Autodesk Inventor part; units mm, degrees
(part 2 of 2)
sketch "スケッチ6" plane through (2.9, 8.6756, -79.5656) normal (1, 0, 0) x (0, 0.1072674, -0.9942302)
  arc A0 (-63.7147, -7.4384) -> (-63.7149, 7.2573) centre (-80.0371, -0.0908) ccw projected
  circle A1 centre (-80.87, 51.0359) radius 3.45
  point P0 (-80.0371, -0.0908)
  point P1 (-80.0371, -0.0908)
  dimension "d31" = 6.9
  constraints: 1 centre point
  measures "d31" diameter of A1
extrude "押し出し5" cut sketch "スケッチ6" against normal blind 10
pattern_circular "円形状パターン3" count 6 over 360 about axis through (35.15, 0, 0) along (1, 0, 0) of "押し出し5"
sketch "スケッチ8" plane through (2.9, 8.6756, -79.5656) normal (1, 0, 0) x (0, 0.1072674, -0.9942302)
  circle A0 centre (-80.0371, -0.0908) radius 22.9
  circle A1 centre (-36.1766, 26.1938) radius 3.45 projected
  circle A2 centre (-35.3437, -24.9328) radius 3.45 projected
  circle A3 centre (-79.2043, -51.2174) radius 3.45 projected
  circle A4 centre (-123.8977, -26.3754) radius 3.45 projected
  circle A5 centre (-124.7305, 24.7513) radius 3.45 projected
  circle A6 centre (-80.87, 51.0359) radius 3.45 projected
  arc A7 (-96.3596, 7.2569) -> (-96.3594, -7.4389) centre (-80.0371, -0.0908) ccw projected
  arc A8 (-96.3596, 7.2569) -> (-94.5619, 10.3707) centre (-95.5391, 8.859) ccw projected
  arc A9 (-81.8351, 17.7187) -> (-94.5619, 10.3707) centre (-80.0371, -0.0908) ccw projected
  arc A10 (-81.8351, 17.7187) -> (-78.2397, 17.7188) centre (-80.0374, 17.8092) ccw projected
  arc A11 (-65.5127, 10.3711) -> (-78.2397, 17.7188) centre (-80.0371, -0.0908) ccw projected
  arc A12 (-65.5127, 10.3711) -> (-63.7149, 7.2573) centre (-64.5354, 8.8595) ccw projected
  arc A13 (-63.7147, -7.4384) -> (-63.7149, 7.2573) centre (-80.0371, -0.0908) ccw projected
  arc A14 (-63.7147, -7.4384) -> (-65.5124, -10.5522) centre (-64.5352, -9.0405) ccw projected
  arc A15 (-78.2392, -17.9002) -> (-65.5124, -10.5522) centre (-80.0371, -0.0908) ccw projected
  arc A16 (-78.2392, -17.9002) -> (-81.8346, -17.9003) centre (-80.0369, -17.9908) ccw projected
  arc A17 (-94.5616, -10.5526) -> (-81.8346, -17.9003) centre (-80.0371, -0.0908) ccw projected
  arc A18 (-94.5616, -10.5526) -> (-96.3594, -7.4389) centre (-95.5389, -9.041) ccw projected
  line L0 (-1.0768, -4.9175) -> (1.1501, -3.6267) projected
  arc A19 (1.1501, -3.6267) -> (1.1812, -2.8194) centre (-80.0371, -0.0908) ccw projected
  line L1 (1.1812, -2.8194) -> (-0.9369, -1.3582) projected
  arc A20 (-0.9369, 1.3582) -> (-0.9369, -1.3582) centre (0, 0) ccw projected
  line L2 (-0.9369, 1.3582) -> (1.1751, 2.8151) projected
  arc A21 (1.1751, 2.8151) -> (1.1417, 3.6315) centre (-80.0371, -0.0908) ccw projected
  line L3 (1.1417, 3.6315) -> (-1.0768, 4.9175) projected
  arc A22 (-1.2899, 7.6255) -> (-1.0768, 4.9175) centre (-0.2493, 6.345) ccw projected
  line L4 (-1.2899, 7.6255) -> (0.6902, 9.2346) projected
  arc A23 (0.6902, 9.2346) -> (0.5904, 10.0614) centre (-80.0371, -0.0908) ccw projected
  line L5 (0.5904, 10.0614) -> (-1.7086, 11.1628) projected
  arc A24 (-2.1335, 13.8457) -> (-1.7086, 11.1628) centre (-0.9956, 12.6509) ccw projected
  line L6 (-2.1335, 13.8457) -> (-0.3005, 15.5913) projected
  arc A25 (-0.3005, 15.5913) -> (-0.4698, 16.4293) centre (-80.0371, -0.0908) ccw projected
  line L7 (-0.4698, 16.4293) -> (-2.8284, 17.3393) projected
  arc A26 (-3.4625, 19.9807) -> (-2.8284, 17.3393) centre (-2.2344, 18.8787) ccw projected
  line L8 (-3.4625, 19.9807) -> (-1.7896, 21.8452) projected
  arc A27 (-1.7896, 21.8452) -> (-2.0327, 22.6945) centre (-80.0371, -0.0908) ccw projected
  line L9 (-2.0327, 22.6945) -> (-4.4294, 23.409) projected
  arc A28 (-5.2688, 25.9924) -> (-4.4294, 23.409) centre (-3.9581, 24.9902) ccw projected
  line L10 (-5.2688, 25.9924) -> (-3.7667, 27.9571) projected
  arc A29 (-3.7667, 27.9571) -> (-4.0884, 28.8169) centre (-80.0371, -0.0908) ccw projected
  line L11 (-4.0884, 28.8169) -> (-6.5017, 29.3343) projected
  arc A30 (-7.5412, 31.8439) -> (-6.5017, 29.3343) centre (-6.1559, 30.9476) ccw projected
  line L12 (-7.5412, 31.8439) -> (-6.2182, 33.889) projected
  arc A31 (-6.2182, 33.889) -> (-6.6241, 34.7574) centre (-80.0371, -0.0908) ccw projected
  line L13 (-6.6241, 34.7574) -> (-9.0325, 35.0787) projected
  arc A32 (-10.2657, 37.499) -> (-9.0325, 35.0787) centre (-8.8143, 36.7142) ccw projected
  line L14 (-10.2657, 37.499) -> (-9.1275, 39.6041) projected
  arc A33 (-9.1275, 39.6041) -> (-9.6237, 40.4779) centre (-80.0371, -0.0908) ccw projected
  line L15 (-9.6237, 40.4779) -> (-12.0062, 40.6069) projected
  arc A34 (-13.4255, 42.923) -> (-12.0062, 40.6069) centre (-11.917, 42.2545) ccw projected
  line L16 (-13.4255, 42.923) -> (-12.4752, 45.0673) projected
  arc A35 (-12.4752, 45.0673) -> (-13.068, 45.9418) centre (-80.0371, -0.0908) ccw projected
  line L17 (-13.068, 45.9418) -> (-15.4045, 45.8847) projected
  arc A36 (-17.0011, 48.0823) -> (-15.4045, 45.8847) centre (-15.4448, 47.5342) ccw projected
  line L18 (-17.0011, 48.0823) -> (-16.2394, 50.2452) projected
  arc A37 (-16.2394, 50.2452) -> (-16.9348, 51.1144) centre (-80.0371, -0.0908) ccw projected
  line L19 (-16.9348, 51.1144) -> (-19.2063, 50.8796) projected
  arc A38 (-20.9705, 52.9451) -> (-19.2063, 50.8796) centre (-19.376, 52.5209) ccw projected
  line L20 (-20.9705, 52.9451) -> (-20.3954, 55.1064) projected
  arc A39 (-20.3954, 55.1064) -> (-21.1994, 55.9626) centre (-80.0371, -0.0908) ccw projected
  line L21 (-21.1994, 55.9626) -> (-23.3884, 55.5608) projected
  arc A40 (-25.3092, 57.4816) -> (-23.3884, 55.5608) centre (-23.6863, 57.1837) ccw projected
  line L22 (-25.3092, 57.4816) -> (-24.9164, 59.6216) projected
  arc A41 (-24.9164, 59.6216) -> (-25.8341, 60.4559) centre (-80.0371, -0.0908) ccw projected
  line L23 (-25.8341, 60.4559) -> (-27.9249, 59.8995) projected
  arc A42 (-29.9904, 61.6637) -> (-27.9249, 59.8995) centre (-28.3491, 61.494) ccw projected
  line L24 (-29.9904, 61.6637) -> (-29.7733, 63.7639) projected
  arc A43 (-29.7733, 63.7639) -> (-30.809, 64.5657) centre (-80.0371, -0.0908) ccw projected
  line L25 (-30.809, 64.5657) -> (-32.7877, 63.8689) projected
  arc A44 (-34.9853, 65.4655) -> (-32.7877, 63.8689) centre (-33.3358, 65.4252) ccw projected
  line L26 (-34.9853, 65.4655) -> (-34.9354, 67.5088) projected
  arc A45 (-34.9354, 67.5088) -> (-36.0922, 68.2665) centre (-80.0371, -0.0908) ccw projected
  line L27 (-36.0922, 68.2665) -> (-37.947, 67.4445) projected
  arc A46 (-40.2631, 68.8638) -> (-37.947, 67.4445) centre (-38.6155, 68.953) ccw projected
  line L28 (-40.2631, 68.8638) -> (-40.3698, 70.8343) projected
  arc A47 (-40.3698, 70.8343) -> (-41.6496, 71.5351) centre (-80.0371, -0.0908) ccw projected
  line L29 (-41.6496, 71.5351) -> (-43.371, 70.6043) projected
  arc A48 (-45.7913, 71.8375) -> (-43.371, 70.6043) centre (-44.1558, 72.0557) ccw projected
  line L30 (-45.7913, 71.8375) -> (-46.0427, 73.7214) projected
  arc A49 (-46.0427, 73.7214) -> (-47.4454, 74.3514) centre (-80.0371, -0.0908) ccw projected
  line L31 (-47.4454, 74.3514) -> (-49.0261, 73.3288) projected
  arc A50 (-51.5357, 74.3683) -> (-49.0261, 73.3288) centre (-49.9224, 74.7141) ccw projected
  line L32 (-51.5357, 74.3683) -> (-51.9185, 76.1536) projected
  arc A51 (-51.9185, 76.1536) -> (-53.4424, 76.6985) centre (-80.0371, -0.0908) ccw projected
  line L33 (-53.4424, 76.6985) -> (-54.8776, 75.6012) projected
  arc A52 (-57.461, 76.4406) -> (-54.8776, 75.6012) centre (-55.8798, 76.9119) ccw projected
  line L34 (-57.461, 76.4406) -> (-57.9609, 78.1173) projected
  arc A53 (-57.9609, 78.1173) -> (-59.6024, 78.5622) centre (-80.0371, -0.0908) ccw projected
  line L35 (-59.6024, 78.5622) -> (-60.8893, 77.4075) projected
  arc A54 (-63.5307, 78.0416) -> (-60.8893, 77.4075) centre (-61.9913, 78.6356) ccw projected
  line L36 (-63.5307, 78.0416) -> (-64.1327, 79.6019) projected
  arc A55 (-64.1327, 79.6019) -> (-65.886, 79.9318) centre (-80.0371, -0.0908) ccw projected
  line L37 (-65.886, 79.9318) -> (-67.0243, 78.7365) projected
  arc A56 (-69.7072, 79.1614) -> (-67.0243, 78.7365) centre (-68.2191, 79.8744) ccw projected
  line L38 (-69.7072, 79.1614) -> (-70.3962, 80.5995) projected
  arc A57 (-70.3962, 80.5995) -> (-72.2514, 80.7996) centre (-80.0371, -0.0908) ccw projected
  line L39 (-72.2514, 80.7996) -> (-73.2346, 79.5639) projected
  arc A58 (-75.9446, 79.749) -> (-73.2346, 79.5639) centre (-74.5257, 80.5912) ccw projected
  line L40 (-75.9446, 79.749) -> (-76.7506, 81.1069) projected
  arc A59 (-76.7506, 81.1069) -> (-78.622, 81.1611) centre (-80.0371, -0.0908) ccw projected
  line L41 (-78.622, 81.1611) -> (-79.5052, 79.8521) projected
  arc A60 (-82.2214, 79.824) -> (-79.5052, 79.8521) centre (-80.873, 80.7749) ccw projected
  line L42 (-82.2214, 79.824) -> (-83.1315, 81.1145) projected
  arc A61 (-83.1315, 81.1145) -> (-85.0013, 81.0217) centre (-80.0371, -0.0908) ccw projected
  line L43 (-85.0013, 81.0217) -> (-85.7791, 79.6474) projected
  arc A62 (-88.4847, 79.4063) -> (-85.7791, 79.6474) centre (-87.215, 80.4601) ccw projected
  line L44 (-88.4847, 79.4063) -> (-89.4932, 80.6214) projected
  arc A63 (-89.4932, 80.6214) -> (-91.35, 80.3821) centre (-80.0371, -0.0908) ccw projected
  line L45 (-91.35, 80.3821) -> (-92.0175, 78.9511) projected
  arc A64 (-94.6959, 78.4984) -> (-92.0175, 78.9511) centre (-93.5129, 79.6486) ccw projected
  line L46 (-94.6959, 78.4984) -> (-95.7967, 79.6307) projected
  arc A65 (-95.7967, 79.6307) -> (-97.629, 79.2465) centre (-80.0371, -0.0908) ccw projected
  line L47 (-97.629, 79.2465) -> (-98.1822, 77.7674) projected
  arc A66 (-100.8168, 77.106) -> (-98.1822, 77.7674) centre (-99.7276, 78.3455) ccw projected
  line L48 (-100.8168, 77.106) -> (-102.0029, 78.1484) projected
  arc A67 (-102.0029, 78.1484) -> (-103.7995, 77.6217) centre (-80.0371, -0.0908) ccw projected
  line L49 (-103.7995, 77.6217) -> (-104.2349, 76.1038) projected
  arc A68 (-106.8095, 75.2377) -> (-104.2349, 76.1038) centre (-105.8209, 76.5588) ccw projected
  line L50 (-106.8095, 75.2377) -> (-108.0738, 76.1838) projected
  arc A69 (-108.0738, 76.1838) -> (-109.8235, 75.5177) centre (-80.0371, -0.0908) ccw projected
  line L51 (-109.8235, 75.5177) -> (-110.1385, 73.9704) projected
  arc A70 (-112.6372, 72.905) -> (-110.1385, 73.9704) centre (-111.7553, 74.2995) ccw projected
  line L52 (-112.6372, 72.905) -> (-113.9718, 73.749) projected
  arc A71 (-113.9718, 73.749) -> (-115.6638, 72.9476) centre (-80.0371, -0.0908) ccw projected
  line L53 (-115.6638, 72.9476) -> (-115.8564, 71.3803) projected
  arc A72 (-118.2639, 70.1222) -> (-115.8564, 71.3803) centre (-117.4941, 71.5816) ccw projected
  line L54 (-118.2639, 70.1222) -> (-119.6606, 70.8589) projected
  arc A73 (-119.6606, 70.8589) -> (-121.2845, 69.9273) centre (-80.0371, -0.0908) ccw projected
  line L55 (-121.2845, 69.9273) -> (-121.3536, 68.3497) projected
  arc A74 (-123.6549, 66.9065) -> (-121.3536, 68.3497) centre (-123.002, 68.4219) ccw projected
  line L56 (-123.6549, 66.9065) -> (-125.1051, 67.5313) projected
  arc A75 (-125.1051, 67.5313) -> (-126.6509, 66.4752) centre (-80.0371, -0.0908) ccw projected
  line L57 (-126.6509, 66.4752) -> (-126.596, 64.897) projected
  arc A76 (-128.777, 63.2778) -> (-126.596, 64.897) centre (-128.245, 64.8397) ccw projected
  line L58 (-128.777, 63.2778) -> (-130.2717, 63.7869) projected
  arc A77 (-130.2717, 63.7869) -> (-131.7299, 62.6127) centre (-80.0371, -0.0908) ccw projected
  line L59 (-131.7299, 62.6127) -> (-131.5514, 61.0437) projected
  arc A78 (-133.5986, 59.2583) -> (-131.5514, 61.0437) centre (-133.1908, 60.8572) ccw projected
  line L60 (-133.5986, 59.2583) -> (-135.1287, 59.6486) projected
  arc A79 (-135.1287, 59.6486) -> (-136.4902, 58.3636) centre (-80.0371, -0.0908) ccw projected
  line L61 (-136.4902, 58.3636) -> (-136.1891, 56.8135) projected
  arc A80 (-138.0899, 54.873) -> (-136.1891, 56.8135) centre (-137.8088, 56.4989) ccw projected
  line L62 (-138.0899, 54.873) -> (-139.6459, 55.142) projected
  arc A81 (-139.6459, 55.142) -> (-140.9025, 53.7542) centre (-80.0371, -0.0908) ccw projected
  line L63 (-140.9025, 53.7542) -> (-140.4807, 52.2325) projected
  arc A82 (-142.2234, 50.1488) -> (-140.4807, 52.2325) centre (-142.0707, 51.7917) ccw projected
  line L64 (-142.2234, 50.1488) -> (-143.7957, 50.2949) projected
  arc A83 (-143.7957, 50.2949) -> (-144.9395, 48.8128) centre (-80.0371, -0.0908) ccw projected
  line L65 (-144.9395, 48.8128) -> (-144.3996, 47.3288) projected
  arc A84 (-145.9734, 45.1149) -> (-144.3996, 47.3288) centre (-145.9501, 46.7647) ccw projected
  line L66 (-145.9734, 45.1149) -> (-147.5524, 45.1371) projected
  arc A85 (-147.5524, 45.1371) -> (-148.5763, 43.5698) centre (-80.0371, -0.0908) ccw projected
  line L67 (-148.5763, 43.5698) -> (-147.9217, 42.1328) projected
  arc A86 (-149.317, 39.8022) -> (-147.9217, 42.1328) centre (-149.4232, 41.4488) ccw projected
  line L68 (-149.317, 39.8022) -> (-150.8928, 39.7005) projected
  arc A87 (-150.8928, 39.7005) -> (-151.7906, 38.0577) centre (-80.0371, -0.0908) ccw projected
  line L69 (-151.7906, 38.0577) -> (-151.0252, 36.6765) projected
  arc A88 (-152.2334, 34.2436) -> (-151.0252, 36.6765) centre (-152.4685, 35.8768) ccw projected
  line L70 (-152.2334, 34.2436) -> (-153.7963, 34.0186) projected
  arc A89 (-153.7963, 34.0186) -> (-154.5625, 32.3104) centre (-80.0371, -0.0908) ccw projected
  line L71 (-154.5625, 32.3104) -> (-153.6911, 30.9935) projected
  arc A90 (-154.7046, 28.4733) -> (-153.6911, 30.9935) centre (-155.0672, 30.083) ccw projected
  line L72 (-154.7046, 28.4733) -> (-156.2452, 28.1264) projected
  arc A91 (-156.2452, 28.1264) -> (-156.8749, 26.3633) centre (-80.0371, -0.0908) ccw projected
  line L73 (-156.8749, 26.3633) -> (-155.9029, 25.1189) projected
  arc A92 (-156.7156, 22.5269) -> (-155.9029, 25.1189) centre (-157.2033, 24.1032) ccw projected
  line L74 (-156.7156, 22.5269) -> (-158.2241, 22.0602) projected
  arc A93 (-158.2241, 22.0602) -> (-158.7136, 20.2532) centre (-80.0371, -0.0908) ccw projected
  line L75 (-158.7136, 20.2532) -> (-157.647, 19.0888) projected
  arc A94 (-158.2538, 16.4411) -> (-157.647, 19.0888) centre (-158.8636, 17.9742) ccw projected
  line L76 (-158.2538, 16.4411) -> (-159.721, 15.8574) projected
  arc A95 (-159.721, 15.8574) -> (-160.0673, 14.0176) centre (-80.0371, -0.0908) ccw projected
  line L77 (-160.0673, 14.0176) -> (-158.9125, 12.9405) projected
  arc A96 (-159.3097, 10.2533) -> (-158.9125, 12.9405) centre (-160.038, 11.7339) ccw projected
  line L78 (-159.3097, 10.2533) -> (-160.7267, 9.5563) projected
  arc A97 (-160.7267, 9.5563) -> (-160.9275, 7.695) centre (-80.0371, -0.0908) ccw projected
  line L79 (-160.9275, 7.695) -> (-159.6918, 6.7118) projected
  arc A98 (-159.8769, 4.0018) -> (-159.6918, 6.7118) centre (-160.7191, 5.4206) ccw projected
  line L80 (-159.8769, 4.0018) -> (-161.2348, 3.1958) projected
  arc A99 (-161.2348, 3.1958) -> (-161.289, 1.3244) centre (-80.0371, -0.0908) ccw projected
  line L81 (-161.289, 1.3244) -> (-159.98, 0.4412) projected
  arc A100 (-159.9519, -2.275) -> (-159.98, 0.4412) centre (-160.9028, -0.9266) ccw projected
  line L82 (-159.9519, -2.275) -> (-161.2424, -3.1851) projected
  arc A101 (-161.2424, -3.1851) -> (-161.1496, -5.0549) centre (-80.0371, -0.0908) ccw projected
  line L83 (-161.1496, -5.0549) -> (-159.7753, -5.8327) projected
  arc A102 (-159.5342, -8.5383) -> (-159.7753, -5.8327) centre (-160.588, -7.2687) ccw projected
  line L84 (-159.5342, -8.5383) -> (-160.7493, -9.5468) projected
  arc A103 (-160.7493, -9.5468) -> (-160.51, -11.4036) centre (-80.0371, -0.0908) ccw projected
  line L85 (-160.51, -11.4036) -> (-159.079, -12.0712) projected
  arc A104 (-158.6263, -14.7495) -> (-159.079, -12.0712) centre (-159.7765, -13.5665) ccw projected
  line L86 (-158.6263, -14.7495) -> (-159.7586, -15.8503) projected
  arc A105 (-159.7586, -15.8503) -> (-159.3744, -17.6826) centre (-80.0371, -0.0908) ccw projected
  line L87 (-159.3744, -17.6826) -> (-157.8953, -18.2358) projected
  arc A106 (-157.234, -20.8704) -> (-157.8953, -18.2358) centre (-158.4734, -19.7812) ccw projected
  line L88 (-157.234, -20.8704) -> (-158.2763, -22.0566) projected
  arc A107 (-158.2763, -22.0566) -> (-157.7496, -23.8531) centre (-80.0371, -0.0908) ccw projected
  line L89 (-157.7496, -23.8531) -> (-156.2317, -24.2885) projected
  arc A108 (-155.3656, -26.8631) -> (-156.2317, -24.2885) centre (-156.6867, -25.8745) ccw projected
  line L90 (-155.3656, -26.8631) -> (-156.3117, -28.1274) projected
  arc A109 (-156.3117, -28.1274) -> (-155.6456, -29.8771) centre (-80.0371, -0.0908) ccw projected
  line L91 (-155.6456, -29.8771) -> (-154.0983, -30.1921) projected
  arc A110 (-153.0329, -32.6908) -> (-154.0983, -30.1921) centre (-154.4274, -31.8089) ccw projected
  line L92 (-153.0329, -32.6908) -> (-153.8769, -34.0254) projected
  arc A111 (-153.8769, -34.0254) -> (-153.0755, -35.7174) centre (-80.0371, -0.0908) ccw projected
  line L93 (-153.0755, -35.7174) -> (-151.5082, -35.9101) projected
  arc A112 (-150.2501, -38.3175) -> (-151.5082, -35.9101) centre (-151.7095, -37.5477) ccw projected
  line L94 (-150.2501, -38.3175) -> (-150.9868, -39.7142) projected
  arc A113 (-150.9868, -39.7142) -> (-150.0552, -41.3381) centre (-80.0371, -0.0908) ccw projected
  line L95 (-150.0552, -41.3381) -> (-148.4776, -41.4072) projected
  arc A114 (-147.0344, -43.7085) -> (-148.4776, -41.4072) centre (-148.5498, -43.0556) ccw projected
  line L96 (-147.0344, -43.7085) -> (-147.6592, -45.1587) projected
  arc A115 (-147.6592, -45.1587) -> (-146.6031, -46.7045) centre (-80.0371, -0.0908) ccw projected
  line L97 (-146.6031, -46.7045) -> (-145.0249, -46.6496) projected
  arc A116 (-143.4057, -48.8306) -> (-145.0249, -46.6496) centre (-144.9676, -48.2986) ccw projected
  line L98 (-143.4057, -48.8306) -> (-143.9148, -50.3254) projected
  arc A117 (-143.9148, -50.3254) -> (-142.7406, -51.7835) centre (-80.0371, -0.0908) ccw projected
  line L99 (-142.7406, -51.7835) -> (-141.1716, -51.605) projected
  arc A118 (-139.3863, -53.6522) -> (-141.1716, -51.605) centre (-140.9851, -53.2444) ccw projected
  line L100 (-139.3863, -53.6522) -> (-139.7765, -55.1823) projected
  arc A119 (-139.7765, -55.1823) -> (-138.4915, -56.5438) centre (-80.0371, -0.0908) ccw projected
  line L101 (-138.4915, -56.5438) -> (-136.9414, -56.2427) projected
  arc A120 (-135.0009, -58.1435) -> (-136.9414, -56.2427) centre (-136.6268, -57.8625) ccw projected
  line L102 (-135.0009, -58.1435) -> (-135.2699, -59.6995) projected
  arc A121 (-135.2699, -59.6995) -> (-133.8821, -60.9561) centre (-80.0371, -0.0908) ccw projected
  line L103 (-133.8821, -60.9561) -> (-132.3604, -60.5343) projected
  arc A122 (-130.2767, -62.277) -> (-132.3604, -60.5343) centre (-131.9196, -62.1243) ccw projected
  line L104 (-130.2767, -62.277) -> (-130.4228, -63.8493) projected
  arc A123 (-130.4228, -63.8493) -> (-128.9407, -64.9931) centre (-80.0371, -0.0908) ccw projected
  line L105 (-128.9407, -64.9931) -> (-127.4567, -64.4532) projected
  arc A124 (-125.2428, -66.027) -> (-127.4567, -64.4532) centre (-126.8926, -66.0038) ccw projected
  line L106 (-125.2428, -66.027) -> (-125.265, -67.606) projected
  arc A125 (-125.265, -67.606) -> (-123.6977, -68.6299) centre (-80.0371, -0.0908) ccw projected
  line L107 (-123.6977, -68.6299) -> (-122.2607, -67.9753) projected
  arc A126 (-119.9301, -69.3706) -> (-122.2607, -67.9753) centre (-121.5767, -69.4768) ccw projected
  line L108 (-119.9301, -69.3706) -> (-119.8284, -70.9464) projected
  arc A127 (-119.8284, -70.9464) -> (-118.1856, -71.8442) centre (-80.0371, -0.0908) ccw projected
  line L109 (-118.1856, -71.8442) -> (-116.8044, -71.0788) projected
  arc A128 (-114.3715, -72.287) -> (-116.8044, -71.0788) centre (-116.0047, -72.5221) ccw projected
  line L110 (-114.3715, -72.287) -> (-114.1465, -73.8499) projected
  arc A129 (-114.1465, -73.8499) -> (-112.4383, -74.6161) centre (-80.0371, -0.0908) ccw projected
  line L111 (-112.4383, -74.6161) -> (-111.1214, -73.7447) projected
  arc A130 (-108.6012, -74.7583) -> (-111.1214, -73.7447) centre (-110.2109, -75.1208) ccw projected
  line L112 (-108.6012, -74.7583) -> (-108.2543, -76.2988) projected
  arc A131 (-108.2543, -76.2988) -> (-106.4912, -76.9286) centre (-80.0371, -0.0908) ccw projected
  line L113 (-106.4912, -76.9286) -> (-105.2468, -75.9565) projected
  arc A132 (-102.6548, -76.7692) -> (-105.2468, -75.9565) centre (-104.2311, -77.2569) ccw projected
  line L114 (-102.6548, -76.7692) -> (-102.1881, -78.2777) projected
  arc A133 (-102.1881, -78.2777) -> (-100.3811, -78.7673) centre (-80.0371, -0.0908) ccw projected
  line L115 (-100.3811, -78.7673) -> (-99.2167, -77.7006) projected
  arc A134 (-96.569, -78.3074) -> (-99.2167, -77.7006) centre (-98.1021, -78.9172) ccw projected
  line L116 (-96.569, -78.3074) -> (-95.9853, -79.7746) projected
  arc A135 (-95.9853, -79.7746) -> (-94.1455, -80.1209) centre (-80.0371, -0.0908) ccw projected
  line L117 (-94.1455, -80.1209) -> (-93.0684, -78.9662) projected
  arc A136 (-90.3812, -79.3633) -> (-93.0684, -78.9662) centre (-91.8618, -80.0916) ccw projected
  line L118 (-90.3812, -79.3633) -> (-89.6842, -80.7803) projected
  arc A137 (-89.6842, -80.7803) -> (-87.8229, -80.9811) centre (-80.0371, -0.0908) ccw projected
  line L119 (-87.8229, -80.9811) -> (-86.8397, -79.7454) projected
  arc A138 (-84.1297, -79.9306) -> (-86.8397, -79.7454) centre (-85.5485, -80.7727) ccw projected
  line L120 (-84.1297, -79.9306) -> (-83.3237, -81.2885) projected
  arc A139 (-83.3237, -81.2885) -> (-81.4523, -81.3426) centre (-80.0371, -0.0908) ccw projected
  line L121 (-81.4523, -81.3426) -> (-80.5691, -80.0336) projected
  arc A140 (-77.8529, -80.0055) -> (-80.5691, -80.0336) centre (-79.2013, -80.9564) ccw projected
  line L122 (-77.8529, -80.0055) -> (-76.9428, -81.296) projected
  arc A141 (-76.9428, -81.296) -> (-75.073, -81.2032) centre (-80.0371, -0.0908) ccw projected
  line L123 (-75.073, -81.2032) -> (-74.2952, -79.8289) projected
  arc A142 (-71.5896, -79.5878) -> (-74.2952, -79.8289) centre (-72.8593, -80.6416) ccw projected
  line L124 (-71.5896, -79.5878) -> (-70.5811, -80.8029) projected
  arc A143 (-70.5811, -80.8029) -> (-68.7243, -80.5636) centre (-80.0371, -0.0908) ccw projected
  line L125 (-68.7243, -80.5636) -> (-68.0568, -79.1326) projected
  arc A144 (-65.3784, -78.68) -> (-68.0568, -79.1326) centre (-66.5614, -79.8301) ccw projected
  line L126 (-65.3784, -78.68) -> (-64.2776, -79.8122) projected
  arc A145 (-64.2776, -79.8122) -> (-62.4453, -79.428) centre (-80.0371, -0.0908) ccw projected
  line L127 (-62.4453, -79.428) -> (-61.8921, -77.949) projected
  arc A146 (-59.2575, -77.2876) -> (-61.8921, -77.949) centre (-60.3467, -78.527) ccw projected
  line L128 (-59.2575, -77.2876) -> (-58.0714, -78.3299) projected
  arc A147 (-58.0714, -78.3299) -> (-56.2748, -77.8032) centre (-80.0371, -0.0908) ccw projected
  line L129 (-56.2748, -77.8032) -> (-55.8394, -76.2853) projected
  arc A148 (-53.2648, -75.4192) -> (-55.8394, -76.2853) centre (-54.2534, -76.7403) ccw projected
  line L130 (-53.2648, -75.4192) -> (-52.0005, -76.3653) projected
  arc A149 (-52.0005, -76.3653) -> (-50.2508, -75.6992) centre (-80.0371, -0.0908) ccw projected
  line L131 (-50.2508, -75.6992) -> (-49.9358, -74.1519) projected
  arc A150 (-47.4371, -73.0865) -> (-49.9358, -74.1519) centre (-48.319, -74.4811) ccw projected
  line L132 (-47.4371, -73.0865) -> (-46.1025, -73.9305) projected
  arc A151 (-46.1025, -73.9305) -> (-44.4105, -73.1292) centre (-80.0371, -0.0908) ccw projected
  line L133 (-44.4105, -73.1292) -> (-44.2178, -71.5619) projected
  arc A152 (-41.8104, -70.3037) -> (-44.2178, -71.5619) centre (-42.5802, -71.7632) ccw projected
  line L134 (-41.8104, -70.3037) -> (-40.4137, -71.0404) projected
  arc A153 (-40.4137, -71.0404) -> (-38.7898, -70.1088) centre (-80.0371, -0.0908) ccw projected
  line L135 (-38.7898, -70.1088) -> (-38.7207, -68.5312) projected
  arc A154 (-36.4194, -67.088) -> (-38.7207, -68.5312) centre (-37.0723, -68.6034) ccw projected
  line L136 (-36.4194, -67.088) -> (-34.9692, -67.7128) projected
  arc A155 (-34.9692, -67.7128) -> (-33.4234, -66.6567) centre (-80.0371, -0.0908) ccw projected
  line L137 (-33.4234, -66.6567) -> (-33.4783, -65.0786) projected
  arc A156 (-31.2973, -63.4593) -> (-33.4783, -65.0786) centre (-31.8293, -65.0212) ccw projected
  line L138 (-31.2973, -63.4593) -> (-29.8026, -63.9684) projected
  arc A157 (-29.8026, -63.9684) -> (-28.3444, -62.7942) centre (-80.0371, -0.0908) ccw projected
  line L139 (-28.3444, -62.7942) -> (-28.5229, -61.2253) projected
  arc A158 (-26.4757, -59.4399) -> (-28.5229, -61.2253) centre (-26.8835, -61.0387) ccw projected
  line L140 (-26.4757, -59.4399) -> (-24.9456, -59.8301) projected
  arc A159 (-24.9456, -59.8301) -> (-23.5841, -58.5452) centre (-80.0371, -0.0908) ccw projected
  line L141 (-23.5841, -58.5452) -> (-23.8852, -56.995) projected
  arc A160 (-21.9844, -55.0545) -> (-23.8852, -56.995) centre (-22.2655, -56.6804) ccw projected
  line L142 (-21.9844, -55.0545) -> (-20.4284, -55.3235) projected
  arc A161 (-20.4284, -55.3235) -> (-19.1718, -53.9357) centre (-80.0371, -0.0908) ccw projected
  line L143 (-19.1718, -53.9357) -> (-19.5936, -52.414) projected
  arc A162 (-17.8509, -50.3303) -> (-19.5936, -52.414) centre (-18.0036, -51.9733) ccw projected
  line L144 (-17.8509, -50.3303) -> (-16.2786, -50.4764) projected
  arc A163 (-16.2786, -50.4764) -> (-15.1348, -48.9943) centre (-80.0371, -0.0908) ccw projected
  line L145 (-15.1348, -48.9943) -> (-15.6747, -47.5104) projected
  arc A164 (-14.1009, -45.2964) -> (-15.6747, -47.5104) centre (-14.1242, -46.9462) ccw projected
  line L146 (-14.1009, -45.2964) -> (-12.5219, -45.3187) projected
  arc A165 (-12.5219, -45.3187) -> (-11.498, -43.7514) centre (-80.0371, -0.0908) ccw projected
  line L147 (-11.498, -43.7514) -> (-12.1526, -42.3144) projected
  arc A166 (-10.7573, -39.9837) -> (-12.1526, -42.3144) centre (-10.6511, -41.6303) ccw projected
  line L148 (-10.7573, -39.9837) -> (-9.1815, -39.8821) projected
  arc A167 (-9.1815, -39.8821) -> (-8.2837, -38.2392) centre (-80.0371, -0.0908) ccw projected
  line L149 (-8.2837, -38.2392) -> (-9.0491, -36.858) projected
  arc A168 (-7.8409, -34.4251) -> (-9.0491, -36.858) centre (-7.6058, -36.0583) ccw projected
  line L150 (-7.8409, -34.4251) -> (-6.278, -34.2001) projected
  arc A169 (-6.278, -34.2001) -> (-5.5118, -32.4919) centre (-80.0371, -0.0908) ccw projected
  line L151 (-5.5118, -32.4919) -> (-6.3832, -31.175) projected
  arc A170 (-5.3697, -28.6548) -> (-6.3832, -31.175) centre (-5.0071, -30.2645) ccw projected
  line L152 (-5.3697, -28.6548) -> (-3.8291, -28.3079) projected
  arc A171 (-3.8291, -28.3079) -> (-3.1993, -26.5449) centre (-80.0371, -0.0908) ccw projected
  line L153 (-3.1993, -26.5449) -> (-4.1714, -25.3004) projected
  arc A172 (-3.3587, -22.7084) -> (-4.1714, -25.3004) centre (-2.871, -24.2847) ccw projected
  line L154 (-3.3587, -22.7084) -> (-1.8502, -22.2417) projected
  arc A173 (-1.8502, -22.2417) -> (-1.3606, -20.4347) centre (-80.0371, -0.0908) ccw projected
  line L155 (-1.3606, -20.4347) -> (-2.4273, -19.2703) projected
  arc A174 (-1.8205, -16.6226) -> (-2.4273, -19.2703) centre (-1.2107, -18.1558) ccw projected
  line L156 (-1.8205, -16.6226) -> (-0.3533, -16.0389) projected
  arc A175 (-0.3533, -16.0389) -> (-0.007, -14.1991) centre (-80.0371, -0.0908) ccw projected
  line L157 (-0.007, -14.1991) -> (-1.1618, -13.122) projected
  arc A176 (-0.7646, -10.4348) -> (-1.1618, -13.122) centre (-0.0363, -11.9154) ccw projected
  line L158 (-0.7646, -10.4348) -> (0.6524, -9.7379) projected
  arc A177 (0.6524, -9.7379) -> (0.8532, -7.8765) centre (-80.0371, -0.0908) ccw projected
  line L159 (0.8532, -7.8765) -> (-0.3825, -6.8933) projected
  arc A178 (-1.0768, -4.9175) -> (-0.3825, -6.8933) centre (0.4734, -5.4827) ccw projected
  dimension "d43" = 45.8
  constraints: 1 centre point, 1 coincident
  measures "d43" diameter of A0
extrude "押し出し7" cut sketch "スケッチ8" against normal blind 0.15 contours A0
sketch "スケッチ9" plane through (2.9, 8.6756, -79.5656) normal (1, 0, 0) x (0, 0.1072674, -0.9942302)
  circle A0 centre (-80.0371, -0.0908) radius 26.0177
  circle A1 centre (-80.87, 51.0359) radius 3.45 projected
  circle A2 centre (-36.1766, 26.1938) radius 3.45 projected
  line L0 (-80.87, 51.0359) -> (-36.1766, 26.1938)
  line L1 (-80.0371, -0.0908) -> (-58.5233, 38.6149)
  circle A3 centre (-52.5256, 49.4053) radius 11
  circle A4 centre (-80.0371, -0.0908) radius 22.9 projected
  dimension "d46" = 22
  constraints: 4 end point, 2 centre point, 1 coincident, 1 midpoint
  measures "d46" diameter of A3
extrude "押し出し8" cut sketch "スケッチ9" against normal through all contours A3
pattern_circular "円形状パターン5" count 6 over 360 about axis through (35.15, 0, 0) along (1, 0, 0) of "押し出し8"
extrude "押し出し9" add sketch "スケッチ9" along normal blind 3 contours A0
body "Solid1"
